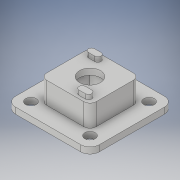
# Autodesk Inventor part: Camera Mount Adapter ODROID plate
Saved by Autodesk Inventor 2019 (Build 230136000, 136)
## iProperties
Created: 2020-10-26
Part Number: Camera Mount Adapter ODROID plate
Material: Generic
Document SubType Name: Modeling
Designer: infinity
Density: 1 g/cm^3
Appearance: Default
Author: infinity
Autodesk Inventor part; units mm, degrees
ref_plane "YZ Plane" through (0, 0, 0) normal (1, 0, 0) x (0, 1, 0)
ref_plane "XZ Plane" through (0, 0, 0) normal (0, 1, 0) x (-1, 0, 0)
ref_plane "XY Plane" through (0, 0, 0) normal (0, 0, 1) x (1, 0, 0)
sketch "Sketch1" plane through (0, 0, 0) normal (0, 1, 0) x (-1, 0, 0)
  line L0 (3, 0) -> (24.05, 0)
  line L1 (27.05, -3) -> (27.05, -24.05)
  line L2 (24.05, -27.05) -> (3, -27.05)
  line L3 (0, -24.05) -> (0, -3)
  line L4 (23.05, -4) -> (4, -4) construction
  line L5 (4, -4) -> (4, -23.05) construction
  line L6 (4, -23.05) -> (23.05, -23.05) construction
  line L7 (23.05, -23.05) -> (23.05, -4) construction
  arc A0 (27.05, -3) -> (24.05, 0) centre (24.05, -3) ccw
  arc A1 (3, 0) -> (0, -3) centre (3, -3) ccw
  arc A2 (0, -24.05) -> (3, -27.05) centre (3, -24.05) ccw
  arc A3 (24.05, -27.05) -> (27.05, -24.05) centre (24.05, -24.05) ccw
  point P0 (0, 0)
  point P1 (27.05, -27.05)
  point P2 (27.05, 0)
  point P3 (0, -27.05)
  dimension "d0" = 19.05
  dimension "d1" = 27.05
  dimension "d2" = 4
  dimension "d3" = 4
  dimension "d4" = 27.05
  dimension "d5" = 4
  dimension "d6" = 3
  constraints: 16 end point, 8 point on circle, 8 point on line, 8 tangent, 4 centre point, 4 coincident, 4 parallel, 3 equal radius, 2 horizontal, 2 perpendicular
  measures "d0" distance of L6.end L4.start
  measures "d1" distance of point (27.05, 0) point (27.05, -27.05)
  measures "d2" distance between parallel lines of L0 L4
  measures "d3" distance between parallel lines of L1 L7
  measures "d4" distance of point (27.05, -27.05) point (0, -27.05)
  measures "d5" distance between parallel lines of L3 L5
  measures "d6" radius of A0
extrude "Extrusion1" add sketch "Sketch1" along normal blind 9
hole "Hole1" at (-23.05, 0, -4) at (-23.05, 0, -23.05) at (-4, 0, -23.05) at (-4, 0, -4) direction (0, 1, 0) diameter 3.4 end through all clearance for "Flat Head Machine Screw" size "M3" standard "Ansi Metric M Profile"
sketch "Sketch2" plane through (0, 9, 0) normal (0, 1, 0) x (1, 0, 0)
  line L0 (-19.525, 5.525) -> (-7.525, 5.525)
  line L1 (-5.525, 7.525) -> (-5.525, 19.525)
  line L2 (-7.525, 21.525) -> (-19.525, 21.525)
  line L3 (-21.525, 19.525) -> (-21.525, 7.525)
  line L4 (-3, 27.05) -> (-24.05, 27.05) projected
  line L5 (-24.05, 0) -> (-3, 0) projected
  line L6 (-27.05, 24.05) -> (-27.05, 3) projected
  line L7 (-24.05, 0) -> (-3, 0) projected
  arc A0 (-3, 0) -> (0, 3) centre (-3, 3) ccw projected
  line L8 (0, 3) -> (0, 24.05) projected
  arc A1 (0, 24.05) -> (-3, 27.05) centre (-3, 24.05) ccw projected
  line L9 (-3, 27.05) -> (-24.05, 27.05) projected
  arc A2 (-24.05, 27.05) -> (-27.05, 24.05) centre (-24.05, 24.05) ccw projected
  line L10 (-27.05, 24.05) -> (-27.05, 3) projected
  arc A3 (-27.05, 3) -> (-24.05, 0) centre (-24.05, 3) ccw projected
  arc A4 (-7.525, 5.525) -> (-5.525, 7.525) centre (-7.525, 7.525) ccw
  arc A5 (-5.525, 19.525) -> (-7.525, 21.525) centre (-7.525, 19.525) ccw
  arc A6 (-19.525, 21.525) -> (-21.525, 19.525) centre (-19.525, 19.525) ccw
  arc A7 (-21.525, 7.525) -> (-19.525, 5.525) centre (-19.525, 7.525) ccw
  point P0 (0, 0)
  point P1 (-21.525, 5.525)
  point P2 (-5.525, 21.525)
  point P3 (-5.525, 5.525)
  point P4 (-21.525, 21.525)
  dimension "d9" = 16
  dimension "d10" = 16
  dimension "d11" = 27.05
  dimension "d12" = 5.525
  dimension "d13" = 5.525
  dimension "d23" = 2
  constraints: 8 end point, 8 point on circle, 8 point on line, 8 tangent, 4 centre point, 3 equal radius, 2 parallel, 1 horizontal, 1 perpendicular
  measures "d9" distance of point (-21.525, 21.525) point (-21.525, 5.525)
  measures "d10" distance of point (-21.525, 5.525) point (-5.525, 5.525)
  measures "d11" distance between parallel lines of L4 L5
  measures "d12" distance between parallel lines of L5 L0
  measures "d13" distance between parallel lines of L6 L3
  measures "d23" radius of A4
extrude "Extrusion2" cut sketch "Sketch2" against normal blind 7
shell "Shell1" thickness 2 removed faces 1 at (-10.7258, 0, -10.7742)
sketch "Sketch3" plane through (0, 9, 0) normal (0, 1, 0) x (1, 0, 0)
  line L0 (-3, 0) -> (-24.05, 0) projected
  line L1 (-27.05, 3) -> (-27.05, 24.05) projected
  line L2 (-10.05, 7.525) -> (-8, 7.525) construction
  line L3 (-10.05, 8.55) -> (-8, 8.55)
  line L4 (-8, 6.5) -> (-10.05, 6.5)
  arc A0 (-10.05, 8.55) -> (-10.05, 6.5) centre (-10.05, 7.525) ccw
  arc A1 (-8, 6.5) -> (-8, 8.55) centre (-8, 7.525) ccw
  line L5 (-17, 19.525) -> (-19.05, 19.525) construction
  line L6 (-17, 20.55) -> (-19.05, 20.55)
  line L7 (-19.05, 18.5) -> (-17, 18.5)
  arc A2 (-17, 18.5) -> (-17, 20.55) centre (-17, 19.525) ccw
  arc A3 (-19.05, 20.55) -> (-19.05, 18.5) centre (-19.05, 19.525) ccw
  point P0 (0, 0)
  point P1 (-13.525, 13.525)
  point P2 (-13.525, 13.525)
  point P3 (-9.025, 7.525)
  point P4 (-18.025, 19.525)
  dimension "d28" = 13.525
  dimension "d29" = 13.525
  dimension "d30" = 2.05
  dimension "d31" = 2.05
  dimension "d32" = 2.05
  dimension "d33" = 2.05
  dimension "d34" = 12
  dimension "d35" = 6
  dimension "d36" = 9
  dimension "d37" = 4.5
  constraints: 16 end point, 8 point on circle, 8 tangent, 4 centre point, 3 parallel, 2 midpoint, 1 coincident, 1 horizontal
  measures "d28" distance from line of L0 point (-13.525, 13.525)
  measures "d29" distance from line of L1 point (-13.525, 13.525)
  measures "d30" distance of L5.start L5.end
  measures "d31" distance of L2.start L2.end
  measures "d32" distance between parallel lines of L4 L3
  measures "d33" distance between parallel lines of L7 L6
  measures "d34" distance between parallel lines of L2 L5
  measures "d35" distance from line of point (-13.525, 13.525) L2
  measures "d36" horizontal distance of point (-18.025, 19.525) point (-9.025, 7.525)
  measures "d37" horizontal distance of point (-9.025, 7.525) point (-13.525, 13.525)
extrude "Extrusion3" add sketch "Sketch3" along normal blind 1.5
hole "Hole2" at (-13.525, 9, -13.525) direction (0, -1, 0) diameter 6.756 end through all clearance for "Flat Head Machine Screw (82)" size "1/4" standard "Ansi Unified Screw Threads"
equation "\"d2\" = -0.5 * d0 + 0.5 * d1"
equation "\"d3\" = d2"
equation "\"d4\" = d1"
equation "\"d5\" = d3"
equation "\"d10\" = d9"
equation "\"d12\" = -0.5 * d9 + 0.5 * d11"
equation "\"d13\" = d12"
equation "\"d28\" = 0.5 * d1"
equation "\"d29\" = d28"
equation "\"d31\" = d30"
equation "\"d32\" = d31"
equation "\"d33\" = d30"
equation "\"d35\" = 0.5 * d34"
equation "\"d37\" = 0.5 * d36"
body "Solid1"
